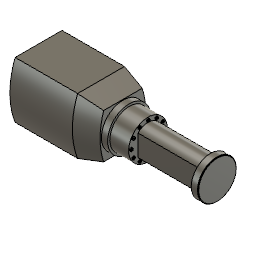
answer (Autodesk Fusion 360 design; units mm, degrees)
part number: 2026-07-30-00-46-47-898
Autodesk Fusion 360 part; units mm, degrees
sketch "Sketch1" plane through (0, 0, 0) normal (1, 0, 0) x (0, 0, -1)
  line L0 (0, 0) -> (0, 45)
  line L1 (0, 0) -> (0, -45)
  line L2 (0, 45) -> (37.5, 45)
  line L3 (0, 45) -> (-37.5, 45)
  line L4 (0, -45) -> (37.5, -45)
  line L5 (0, -45) -> (-37.5, -45)
  arc A0 (-37.5, 45) -> (-37.5, -45) centre (79.119, 0) ccw
  arc A1 (37.5, -45) -> (37.5, 45) centre (-79.119, 0) ccw
  dimension "d1" = 45
  dimension "d2" = 45
  dimension "d3" = 37.5
  dimension "d4" = 37.5
  dimension "d5" = 37.5
  dimension "d6" = 37.5
  dimension "d8" = 125
  constraint coincident L0.start L1.start
  constraint vertical L0
  constraint parallel L0 L1
  constraint perpendicular L0 L2
  constraint perpendicular L0 L3
  constraint perpendicular L1 L4
  constraint perpendicular L1 L5
  constraint symmetric L0 L3.end L2.end
  constraint symmetric L0 L5.end L4.end
  constraint symmetric L0 A0 A1
  measures "d1" distance of L0.start L0.end
  measures "d2" distance of L0.start L1.end
  measures "d3" distance of L0.end L2.end
  measures "d4" distance of L0.end L3.end
  measures "d5" distance of L1.end L4.end
  measures "d6" distance of L1.end L5.end
  measures "d8" radius of A0
extrude "Extrude1" add sketch "Sketch1" along normal blind 100
extrude "Extrude2" add 1 faces at (100, 3.0661, -15.1807) along direction (1, 0, 0) blind 35 draft -15
sketch "Sketch2" plane through (135, 0, 0) normal (1, 0, 0) x (0, 0, -1)
  line L0 (-30.8786, -35.6218) -> (30.8786, -35.6218)
  arc A0 (30.8786, -35.6218) -> (30.8786, 35.6218) centre (-79.119, 0) ccw
  line L1 (30.8786, 35.6218) -> (-30.8786, 35.6218)
  arc A1 (-30.8786, 35.6218) -> (-30.8786, -35.6218) centre (79.119, 0) ccw
  circle A2 centre (0, 0) radius 34.5
  dimension "d13" = 69
  constraint coincident A2.centre origin
  measures "d13" diameter of A2
extrude "Extrude3" add sketch "Sketch2" along normal blind 10 contours A2
sketch "Sketch3" plane through (145, 0, 0) normal (1, 0, 0) x (0, 0, -1)
  circle A0 centre (0, 0) radius 34.5
  circle A1 centre (0, 0) radius 31
  dimension "d16" = 62
  constraint coincident A0.centre A1.centre
  measures "d16" diameter of A1
extrude "Extrude4" add sketch "Sketch3" along normal blind 30 contours A1
sketch "Sketch4" plane through (175, 0, 0) normal (1, 0, 0) x (0, 0, -1)
  circle A0 centre (0, 0) radius 31
  line L0 (0, 0) -> (27, 0)
  circle A1 centre (27, 0) radius 2.5
  circle A2 centre (27, 0) radius 1.5
  dimension "d19" = 27
  dimension "d20" = 5
  dimension "d21" = -1
  constraint coincident A0.centre L0.start
  constraint horizontal L0
  constraint coincident L0.end A1.centre
  measures "d19" distance of A0.centre L0.end
  measures "d20" diameter of A1
extrude "Extrude5" add sketch "Sketch4" along normal blind 1 contours A1
pattern_circular "C-Pattern1" count 12 over 360 about axis through (175, 0, 0) along (1, 0, 0) of "Extrude5"
sketch "Sketch5" plane through (175, 0, 0) normal (1, 0, 0) x (0, 0, -1)
  circle A0 centre (27, 0) radius 2.5
  circle A1 centre (0, 0) radius 31
  circle A2 centre (23.3827, 13.5) radius 2.5
  circle A3 centre (13.5, 23.3827) radius 2.5
  circle A4 centre (0, 27) radius 2.5
  circle A5 centre (-13.5, 23.3827) radius 2.5
  circle A6 centre (-23.3827, 13.5) radius 2.5
  circle A7 centre (-27, 0) radius 2.5
  circle A8 centre (-23.3827, -13.5) radius 2.5
  circle A9 centre (-13.5, -23.3827) radius 2.5
  circle A10 centre (0, -27) radius 2.5
  circle A11 centre (13.5, -23.3827) radius 2.5
  circle A12 centre (23.3827, -13.5) radius 2.5
  line L0 (0, 0) -> (16, 0)
  line L1 (16, 0) -> (16, 17)
  line L2 (16, 0) -> (16, -17)
  line L3 (0, 0) -> (0, -8.0593)
  line L4 (-16, 0) -> (-16, 17)
  line L5 (-16, 0) -> (-16, -17)
  arc A13 (16, 17) -> (-16, 17) centre (0, 1.9003) ccw
  arc A14 (-16, -17) -> (16, -17) centre (0, -1.9003) ccw
  dimension "d26" = 16
  dimension "d27" = 17
  dimension "d28" = 17
  dimension "d29" = 22
  constraint coincident A1.centre L0.start
  constraint horizontal L0
  constraint perpendicular L0 L1
  constraint perpendicular L0 L2
  constraint perpendicular L0 L3
  constraint symmetric L0.end L3 L4.start
  constraint symmetric L1.end L3 L4.end
  constraint symmetric L2.end L3 L5.end
  constraint symmetric L0 L1.end L2.end
  constraint symmetric L0 L4.end L5.end
  constraint symmetric L0 A13 A14
  measures "d26" distance of A1.centre L0.end
  measures "d27" distance of L0.end L1.end
  measures "d28" distance of L0.end L2.end
  measures "d29" radius of A13
extrude "Extrude6" add sketch "Sketch5" along normal blind 100 contours L1 L2 L4 L5 A13 A14
sketch "Sketch6" plane through (275, 0, 0) normal (1, 0, 0) x (0, 0, -1)
  line L0 (-16, 17) -> (-16, -17)
  arc A0 (-16, -17) -> (16, -17) centre (0, -1.9003) ccw
  line L1 (16, -17) -> (16, 17)
  arc A1 (16, 17) -> (-16, 17) centre (0, 1.9003) ccw
  circle A2 centre (0, 0) radius 31
  circle A3 centre (0, 0) radius 30
  dimension "d32" = 62
  dimension "d35" = -1
  constraint coincident A2.centre A3.centre
  measures "d32" diameter of A2
extrude "Extrude7" add sketch "Sketch6" along normal blind 10 contours L0 A0 L1 A1 | A2 | A3
sketch "Sketch7" plane through (285, 0, 0) normal (1, 0, 0) x (0, 0, -1)
  circle A0 centre (0, 0) radius 31
  circle A1 centre (0, 0) radius 30
  dimension "d36" = -1
extrude "Extrude8" add sketch "Sketch7" along normal blind 1 contours A1
